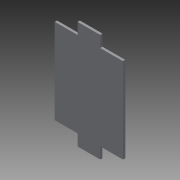
# Autodesk Inventor part: base2
Saved by Autodesk Inventor 2014 SP1 (Build 180222100, 222)
## iProperties
Created: 2014-10-13
Part Number: base2
Material: Générique
Document SubType Name: Modeling
Designer: astralien3000
Density: 1 g/cm^3
Appearance: Par défaut
Author: astralien3000
Autodesk Inventor part; units mm, degrees
ref_plane "YZ Plane" through (0, 0, 0) normal (1, 0, 0) x (0, 1, 0)
ref_plane "XZ Plane" through (0, 0, 0) normal (0, 1, 0) x (-1, 0, 0)
ref_plane "XY Plane" through (0, 0, 0) normal (0, 0, 1) x (1, 0, 0)
sketch "Esquisse1" plane through (0, 0, 0) normal (0, 1, 0) x (-1, 0, 0)
  line L0 (-20, 95) -> (20, 95)
  line L1 (20, 95) -> (20, -95)
  line L2 (20, -95) -> (-20, -95)
  line L3 (-20, -95) -> (-20, 95)
  line L4 (-20, 75) -> (-60, 75)
  line L5 (-60, 75) -> (-60, -75)
  line L6 (-60, -75) -> (-20, -75)
  line L7 (-20, -75) -> (-20, 75)
  line L8 (20, 75) -> (60, 75)
  line L9 (60, 75) -> (60, -75)
  line L10 (60, -75) -> (20, -75)
  line L11 (20, -75) -> (20, 75)
  point P0 (0, 0)
  dimension "d0" = 190
  dimension "d1" = 120
  dimension "d2" = 40
  dimension "d3" = 40
  dimension "d4" = 20
  dimension "d5" = 95
  dimension "d6" = 20
  dimension "d7" = 20
  constraints: 24 end point, 6 parallel, 3 horizontal, 3 perpendicular, 2 collinear, 2 point on line
  measures "d0" distance between parallel lines of L2 L0
  measures "d1" distance between parallel lines of L5 L9
  measures "d2" distance of L1.end L2.end
  measures "d3" distance of L4.start L4.end
  measures "d4" distance from line of point (0, 0) L1
  measures "d5" distance from line of point (0, 0) L2
  measures "d6" distance between parallel lines of L2 L6
  measures "d7" distance between parallel lines of L0 L4
extrude "Extrusion1" add sketch "Esquisse1" along normal blind 4
equation "\"d2\" = d1 - 2 * d3"
equation "\"d4\" = 0.5 * d2"
equation "\"d5\" = 0.5 * d0"
equation "\"d7\" = d6"
